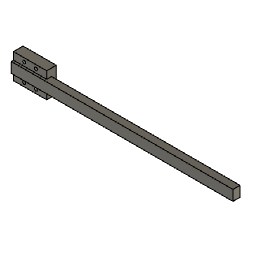
water-suply (Autodesk Fusion 360 archive; units mm, degrees)
design "rail 150mm"
Autodesk Fusion 360 part; units mm, degrees
note: some values were not read from the file. Set by a fixed rule: the direction of a hole.
sketch "스케치1" plane through (0, 0, 0) normal (0, 1, 0) x (1, 0, 0)
  line L0 (0, 0) -> (150, 0) construction
  line L1 (150, 0) -> (150, -17) construction
  line L2 (150, -17) -> (0, -17) construction
  line L3 (0, -17) -> (0, 0) construction
  line L4 (0, -12) -> (150, -12)
  line L5 (150, -12) -> (150, -5)
  line L6 (150, -5) -> (0, -5)
  line L7 (0, -5) -> (0, -12)
  line L8 (35.8106, -17) -> (58.3106, -17)
  line L9 (58.3106, -17) -> (58.3106, 0)
  line L10 (58.3106, 0) -> (35.8106, 0)
  line L11 (35.8106, 0) -> (35.8106, -17)
  line L12 (43.061, -14.5007) -> (51.061, -14.5007) construction
  line L13 (51.061, -14.5007) -> (51.061, -2.5007) construction
  line L14 (51.061, -2.5007) -> (43.061, -2.5007) construction
  line L15 (43.061, -2.5007) -> (43.061, -14.5007) construction
  line L16 (58.3106, -17) -> (35.8106, 0) construction
  line L17 (35.8106, -17) -> (58.3106, 0) construction
  line L18 (47.0606, -8.5) -> (43.061, -2.5007) construction
  line L19 (43.061, -14.5007) -> (47.0606, -8.5) construction
  line L20 (47.0606, -8.5) -> (51.061, -2.5007) construction
  line L21 (51.061, -14.5007) -> (47.0606, -8.5) construction
  point P0 (47.0606, -8.5)
  point P1 (47.0606, -8.5)
  dimension "d1" = 150
  dimension "d2" = 17
  dimension "d3" = 7
  dimension "d4" = 22.5
  dimension "d24" = 8
  dimension "d25" = 12
  constraint horizontal L0
  constraint vertical L1
  constraint horizontal L2
  constraint vertical L3
  constraint coincident L0.start L3.end
  constraint horizontal L4
  constraint vertical L5
  constraint horizontal L6
  constraint vertical L7
  constraint coincident L3 L4.start
  constraint midpoint L3 L7
  constraint horizontal L8
  constraint vertical L9
  constraint horizontal L10
  constraint vertical L11
  constraint coincident L2 L8.start
  constraint collinear L0 L10
  constraint horizontal L12
  constraint vertical L13
  constraint horizontal L14
  constraint vertical L15
  constraint coincident P1 P0
  constraint midpoint L17 P1
  measures "d1" distance of L0.start L0.end
  measures "d2" distance of L0.start L2.end
  measures "d3" distance of L4.start L6.end
  measures "d4" distance of L8.start L8.end
  measures "d24" distance of L12.start L12.end
  measures "d25" distance of L12.start L14.end
extrude "돌출1" add sketch "스케치1" along normal blind 4.8 contours L4 L6 L7 L11 | L4 L6 L9 L11 | L4 L5 L6 L9 makes body 1
copy_body "본체->구성요소1" bodies 1 removing the originals makes body 2 in component "Component'"
extrude "돌출1'" add sketch "스케치1" along normal blind 6.5 from surface at 1.5 separate body contours L4 L6 L9 L11 | L4 L8 L9 L11 | L6 L9 L10 L11 makes body 3 in component "Component"
combine "결합1" operation cut target body 3 tool bodies 2 keep tools in component "Component"
hole "구멍1" at (51.061, 0, 14.5007) at (43.061, 0, 14.5007) at (43.061, 0, 2.5007) at (51.061, 0, 2.5007) direction (0, 1, 0) diameter 2 end through all bodies 3 in component "Component"
component "Component" placed x (1, 0, 0) y (0, 1, 0) z (0, 0, 1) at (-35.8106, 0, 0)
component "Component'" placed x (1, 0, 0) y (0, 1, 0) z (0, 0, 1) at (0, 0, 0)
equation "d21 = -150.00 mm + 22.5 mm"

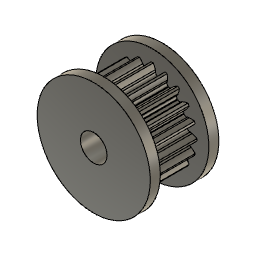
design "gpa20gt2060-a-h4"
description: Spur Gear; Module: 0.611000; Number of Teeth: 20; Pressure Angle: 20.000000; Root Fillet Radius: 0.036000; Clearance: 0.010000; Gear Thickness: 1.030000; Hole Diameter: 0.400000;
Autodesk Fusion 360 part; units mm, degrees
sketch "sketch 251" plane through (0, 0, 0) normal (0, 1, 0) x (1, 0, 0)
  spline S0 degree 3 poles (-6.7198, -0.1571) (-6.4139, -0.333) (-6.1651, -0.4166) (-5.9924, -0.4559) knots 0 0 0 0 1 1 1 1
  spline S1 degree 3 poles (-5.5463, -1.2926) (-5.63, -1.3139) (-5.7122, -1.3421) (-5.84, -1.4181) knots 0 0 0 0 1 1 1 1
  arc A0 (-5.2876, -0.7901) -> (-5.2729, -0.8825) centre (0, 0) ccw
  arc A1 (-5.2876, -0.7901) -> (-5.6742, -0.4846) centre (-5.6436, -0.8433) ccw
  arc A2 (-5.5463, -1.2926) -> (-5.2729, -0.8825) centre (-5.628, -0.942) ccw
  spline S2 degree 3 poles (-6.3424, -2.2259) (-5.9971, -2.2987) (-5.7346, -2.3013) (-5.5582, -2.2853) knots 0 0 0 0 1 1 1 1
  spline S3 degree 3 poles (-5.9924, -0.4559) (-5.8473, -0.4887) (-5.7605, -0.4902) (-5.6742, -0.4846) knots 0 0 0 0 1 1 1 1
  spline S4 degree 3 poles (-5.9924, 0.4559) (-6.1651, 0.4166) (-6.4139, 0.333) (-6.7198, 0.1571) knots 0 0 0 0 1 1 1 1
  arc A3 (-6.7198, 0.1571) -> (-6.7198, -0.1571) centre (0, 0) ccw
  spline S5 degree 3 poles (-5.3441, -4.0769) (-4.9932, -4.0394) (-4.7428, -3.9608) (-4.5799, -3.8911) knots 0 0 0 0 1 1 1 1
  spline S6 degree 3 poles (-3.1534, -5.1159) (-3.0416, -5.0179) (-2.9894, -4.9484) (-2.9432, -4.8754) knots 0 0 0 0 1 1 1 1
  arc A4 (-2.4688, -4.7421) -> (-2.3853, -4.7846) centre (0, 0) ccw
  spline S7 degree 3 poles (-5.5582, -2.2853) (-5.4101, -2.2717) (-5.3271, -2.2463) (-5.2468, -2.2143) knots 0 0 0 0 1 1 1 1
  arc A5 (-3.7273, -4.3057) -> (-3.7471, -3.8133) centre (-3.9994, -4.0701) ccw
  spline S8 degree 3 poles (-2.2853, -5.5582) (-2.3013, -5.7346) (-2.2987, -5.9971) (-2.2259, -6.3424) knots 0 0 0 0 1 1 1 1
  arc A6 (-0.1571, -6.7198) -> (0.1571, -6.7198) centre (0, 0) ccw
  spline S9 degree 3 poles (-3.7273, -4.3057) (-3.7825, -4.3722) (-3.8323, -4.4433) (-3.8911, -4.5799) knots 0 0 0 0 1 1 1 1
  spline S10 degree 3 poles (-0.4559, -5.9924) (-0.4166, -6.1651) (-0.333, -6.4139) (-0.1571, -6.7198) knots 0 0 0 0 1 1 1 1
  spline S11 degree 3 poles (-3.8911, -4.5799) (-3.9608, -4.7428) (-4.0394, -4.9932) (-4.0769, -5.3441) knots 0 0 0 0 1 1 1 1
  spline S12 degree 3 poles (0.1571, -6.7198) (0.333, -6.4139) (0.4166, -6.1651) (0.4559, -5.9924) knots 0 0 0 0 1 1 1 1
  arc A7 (-4.0769, -5.3441) -> (-3.8227, -5.5288) centre (0, 0) ccw
  spline S13 degree 3 poles (-2.2143, -5.2468) (-2.2463, -5.3271) (-2.2717, -5.4101) (-2.2853, -5.5582) knots 0 0 0 0 1 1 1 1
  spline S14 degree 3 poles (1.2926, -5.5463) (1.3139, -5.63) (1.3421, -5.7122) (1.4181, -5.84) knots 0 0 0 0 1 1 1 1
  spline S15 degree 3 poles (0.4559, -5.9924) (0.4887, -5.8473) (0.4902, -5.7605) (0.4846, -5.6742) knots 0 0 0 0 1 1 1 1
  arc A8 (-0.4846, -5.6742) -> (-0.7901, -5.2876) centre (-0.8433, -5.6436) ccw
  spline S16 degree 3 poles (-0.4846, -5.6742) (-0.4902, -5.7605) (-0.4887, -5.8473) (-0.4559, -5.9924) knots 0 0 0 0 1 1 1 1
  arc A9 (-0.8825, -5.2729) -> (-0.7901, -5.2876) centre (0, 0) ccw
  arc A10 (-5.5288, -3.8227) -> (-5.3441, -4.0769) centre (0, 0) ccw
  arc A11 (1.2926, -5.5463) -> (0.8825, -5.2729) centre (0.942, -5.628) ccw
  arc A12 (0.7901, -5.2876) -> (0.8825, -5.2729) centre (0, 0) ccw
  spline S17 degree 3 poles (-5.1159, -3.1534) (-5.2325, -3.2867) (-5.3847, -3.5006) (-5.5288, -3.8227) knots 0 0 0 0 1 1 1 1
  spline S18 degree 3 poles (-5.84, -1.4181) (-5.9921, -1.5089) (-6.2029, -1.6653) (-6.4395, -1.9271) knots 0 0 0 0 1 1 1 1
  arc A13 (-2.4688, -4.7421) -> (-2.9432, -4.8754) centre (-2.635, -5.0614) ccw
  spline S19 degree 3 poles (-3.8227, -5.5288) (-3.5006, -5.3847) (-3.2867, -5.2325) (-3.1534, -5.1159) knots 0 0 0 0 1 1 1 1
  arc A14 (-4.8754, -2.9432) -> (-4.7421, -2.4688) centre (-5.0614, -2.635) ccw
  arc A15 (-2.2259, -6.3424) -> (-1.9271, -6.4395) centre (0, 0) ccw
  spline S20 degree 3 poles (-4.5799, -3.8911) (-4.4433, -3.8323) (-4.3722, -3.7825) (-4.3057, -3.7273) knots 0 0 0 0 1 1 1 1
  arc A16 (-0.8825, -5.2729) -> (-1.2926, -5.5463) centre (-0.942, -5.628) ccw
  spline S21 degree 3 poles (-1.4181, -5.84) (-1.3421, -5.7122) (-1.3139, -5.63) (-1.2926, -5.5463) knots 0 0 0 0 1 1 1 1
  arc A17 (0.7901, -5.2876) -> (0.4846, -5.6742) centre (0.8433, -5.6436) ccw
  spline S22 degree 3 poles (1.4181, -5.84) (1.5089, -5.9921) (1.6653, -6.2029) (1.9271, -6.4395) knots 0 0 0 0 1 1 1 1
  spline S23 degree 3 poles (-4.8754, -2.9432) (-4.9484, -2.9894) (-5.0179, -3.0416) (-5.1159, -3.1534) knots 0 0 0 0 1 1 1 1
  arc A18 (-4.7846, -2.3853) -> (-4.7421, -2.4688) centre (0, 0) ccw
  arc A19 (-3.8133, -3.7471) -> (-4.3057, -3.7273) centre (-4.0701, -3.9994) ccw
  arc A20 (-2.2143, -5.2468) -> (-2.3853, -4.7846) centre (-2.546, -5.1068) ccw
  spline S24 degree 3 poles (-1.9271, -6.4395) (-1.6653, -6.2029) (-1.5089, -5.9921) (-1.4181, -5.84) knots 0 0 0 0 1 1 1 1
  arc A21 (-6.4395, -1.9271) -> (-6.3424, -2.2259) centre (0, 0) ccw
  arc A22 (-4.7846, -2.3853) -> (-5.2468, -2.2143) centre (-5.1068, -2.546) ccw
  arc A23 (-3.8133, -3.7471) -> (-3.7471, -3.8133) centre (0, 0) ccw
  arc A24 (5.3441, -4.0769) -> (5.5288, -3.8227) centre (0, 0) ccw
  arc A25 (2.3853, -4.7846) -> (2.4688, -4.7421) centre (0, 0) ccw
  spline S25 degree 3 poles (4.3057, -3.7273) (4.3722, -3.7825) (4.4433, -3.8323) (4.5799, -3.8911) knots 0 0 0 0 1 1 1 1
  spline S26 degree 3 poles (5.1159, -3.1534) (5.0179, -3.0416) (4.9484, -2.9894) (4.8754, -2.9432) knots 0 0 0 0 1 1 1 1
  arc A26 (1.9271, -6.4395) -> (2.2259, -6.3424) centre (0, 0) ccw
  arc A27 (4.7421, -2.4688) -> (4.8754, -2.9432) centre (5.0614, -2.635) ccw
  arc A28 (5.2468, -2.2143) -> (4.7846, -2.3853) centre (5.1068, -2.546) ccw
  spline S27 degree 3 poles (5.5288, -3.8227) (5.3847, -3.5006) (5.2325, -3.2867) (5.1159, -3.1534) knots 0 0 0 0 1 1 1 1
  arc A29 (2.9432, -4.8754) -> (2.4688, -4.7421) centre (2.635, -5.0614) ccw
  spline S28 degree 3 poles (2.9432, -4.8754) (2.9894, -4.9484) (3.0416, -5.0179) (3.1534, -5.1159) knots 0 0 0 0 1 1 1 1
  arc A30 (3.8227, -5.5288) -> (4.0769, -5.3441) centre (0, 0) ccw
  arc A31 (3.7471, -3.8133) -> (3.8133, -3.7471) centre (0, 0) ccw
  spline S29 degree 3 poles (4.5799, -3.8911) (4.7428, -3.9608) (4.9932, -4.0394) (5.3441, -4.0769) knots 0 0 0 0 1 1 1 1
  arc A32 (4.3057, -3.7273) -> (3.8133, -3.7471) centre (4.0701, -3.9994) ccw
  spline S30 degree 3 poles (3.1534, -5.1159) (3.2867, -5.2325) (3.5006, -5.3847) (3.8227, -5.5288) knots 0 0 0 0 1 1 1 1
  spline S31 degree 3 poles (4.0769, -5.3441) (4.0394, -4.9932) (3.9608, -4.7428) (3.8911, -4.5799) knots 0 0 0 0 1 1 1 1
  arc A33 (4.7421, -2.4688) -> (4.7846, -2.3853) centre (0, 0) ccw
  arc A34 (3.7471, -3.8133) -> (3.7273, -4.3057) centre (3.9994, -4.0701) ccw
  spline S32 degree 3 poles (3.8911, -4.5799) (3.8323, -4.4433) (3.7825, -4.3722) (3.7273, -4.3057) knots 0 0 0 0 1 1 1 1
  spline S33 degree 3 poles (2.2259, -6.3424) (2.2987, -5.9971) (2.3013, -5.7346) (2.2853, -5.5582) knots 0 0 0 0 1 1 1 1
  arc A35 (2.3853, -4.7846) -> (2.2143, -5.2468) centre (2.546, -5.1068) ccw
  spline S34 degree 3 poles (2.2853, -5.5582) (2.2717, -5.4101) (2.2463, -5.3271) (2.2143, -5.2468) knots 0 0 0 0 1 1 1 1
  circle A36 centre (0, 0) radius 2
  spline S35 degree 3 poles (5.2468, -2.2143) (5.3271, -2.2463) (5.4101, -2.2717) (5.5582, -2.2853) knots 0 0 0 0 1 1 1 1
  spline S36 degree 3 poles (-5.84, 1.4181) (-5.7122, 1.3421) (-5.63, 1.3139) (-5.5463, 1.2926) knots 0 0 0 0 1 1 1 1
  arc A37 (-4.7421, 2.4688) -> (-4.8754, 2.9432) centre (-5.0614, 2.635) ccw
  arc A38 (-6.3424, 2.2259) -> (-6.4395, 1.9271) centre (0, 0) ccw
  spline S37 degree 3 poles (-5.5288, 3.8227) (-5.3847, 3.5006) (-5.2325, 3.2867) (-5.1159, 3.1534) knots 0 0 0 0 1 1 1 1
  spline S38 degree 3 poles (-6.4395, 1.9271) (-6.2029, 1.6653) (-5.9921, 1.5089) (-5.84, 1.4181) knots 0 0 0 0 1 1 1 1
  arc A39 (5.2729, -0.8825) -> (5.2876, -0.7901) centre (0, 0) ccw
  arc A40 (5.6742, -0.4846) -> (5.2876, -0.7901) centre (5.6436, -0.8433) ccw
  arc A41 (-5.6742, 0.4846) -> (-5.2876, 0.7901) centre (-5.6436, 0.8433) ccw
  spline S39 degree 3 poles (6.4395, -1.9271) (6.2029, -1.6653) (5.9921, -1.5089) (5.84, -1.4181) knots 0 0 0 0 1 1 1 1
  spline S40 degree 3 poles (5.5582, -2.2853) (5.7346, -2.3013) (5.9971, -2.2987) (6.3424, -2.2259) knots 0 0 0 0 1 1 1 1
  spline S41 degree 3 poles (5.84, -1.4181) (5.7122, -1.3421) (5.63, -1.3139) (5.5463, -1.2926) knots 0 0 0 0 1 1 1 1
  arc A42 (5.2729, -0.8825) -> (5.5463, -1.2926) centre (5.628, -0.942) ccw
  spline S42 degree 3 poles (-5.6742, 0.4846) (-5.7605, 0.4902) (-5.8473, 0.4887) (-5.9924, 0.4559) knots 0 0 0 0 1 1 1 1
  arc A43 (-5.2729, 0.8825) -> (-5.2876, 0.7901) centre (0, 0) ccw
  arc A44 (-5.2729, 0.8825) -> (-5.5463, 1.2926) centre (-5.628, 0.942) ccw
  arc A45 (-4.7421, 2.4688) -> (-4.7846, 2.3853) centre (0, 0) ccw
  arc A46 (6.3424, -2.2259) -> (6.4395, -1.9271) centre (0, 0) ccw
  spline S43 degree 3 poles (-5.5582, 2.2853) (-5.7346, 2.3013) (-5.9971, 2.2987) (-6.3424, 2.2259) knots 0 0 0 0 1 1 1 1
  spline S44 degree 3 poles (-5.2468, 2.2143) (-5.3271, 2.2463) (-5.4101, 2.2717) (-5.5582, 2.2853) knots 0 0 0 0 1 1 1 1
  spline S45 degree 3 poles (-5.1159, 3.1534) (-5.0179, 3.0416) (-4.9484, 2.9894) (-4.8754, 2.9432) knots 0 0 0 0 1 1 1 1
  arc A47 (-5.2468, 2.2143) -> (-4.7846, 2.3853) centre (-5.1068, 2.546) ccw
  arc A48 (3.7273, 4.3057) -> (3.7471, 3.8133) centre (3.9994, 4.0701) ccw
  spline S46 degree 3 poles (5.9924, 0.4559) (5.8473, 0.4887) (5.7605, 0.4902) (5.6742, 0.4846) knots 0 0 0 0 1 1 1 1
  arc A49 (4.7846, 2.3853) -> (4.7421, 2.4688) centre (0, 0) ccw
  spline S47 degree 3 poles (3.1534, 5.1159) (3.0416, 5.0179) (2.9894, 4.9484) (2.9432, 4.8754) knots 0 0 0 0 1 1 1 1
  arc A50 (5.2876, 0.7901) -> (5.6742, 0.4846) centre (5.6436, 0.8433) ccw
  arc A51 (5.5288, 3.8227) -> (5.3441, 4.0769) centre (0, 0) ccw
  spline S48 degree 3 poles (3.8911, 4.5799) (3.9608, 4.7428) (4.0394, 4.9932) (4.0769, 5.3441) knots 0 0 0 0 1 1 1 1
  arc A52 (0.8825, 5.2729) -> (0.7901, 5.2876) centre (0, 0) ccw
  arc A53 (-2.3853, 4.7846) -> (-2.4688, 4.7421) centre (0, 0) ccw
  spline S49 degree 3 poles (-2.2259, 6.3424) (-2.2987, 5.9971) (-2.3013, 5.7346) (-2.2853, 5.5582) knots 0 0 0 0 1 1 1 1
  spline S50 degree 3 poles (-2.9432, 4.8754) (-2.9894, 4.9484) (-3.0416, 5.0179) (-3.1534, 5.1159) knots 0 0 0 0 1 1 1 1
  arc A54 (-2.9432, 4.8754) -> (-2.4688, 4.7421) centre (-2.635, 5.0614) ccw
  arc A55 (5.5463, 1.2926) -> (5.2729, 0.8825) centre (5.628, 0.942) ccw
  spline S51 degree 3 poles (-4.3057, 3.7273) (-4.3722, 3.7825) (-4.4433, 3.8323) (-4.5799, 3.8911) knots 0 0 0 0 1 1 1 1
  arc A56 (-0.7901, 5.2876) -> (-0.4846, 5.6742) centre (-0.8433, 5.6436) ccw
  spline S52 degree 3 poles (-4.0769, 5.3441) (-4.0394, 4.9932) (-3.9608, 4.7428) (-3.8911, 4.5799) knots 0 0 0 0 1 1 1 1
  spline S53 degree 3 poles (1.4181, 5.84) (1.3421, 5.7122) (1.3139, 5.63) (1.2926, 5.5463) knots 0 0 0 0 1 1 1 1
  spline S54 degree 3 poles (5.5463, 1.2926) (5.63, 1.3139) (5.7122, 1.3421) (5.84, 1.4181) knots 0 0 0 0 1 1 1 1
  spline S55 degree 3 poles (5.9924, -0.4559) (6.1651, -0.4166) (6.4139, -0.333) (6.7198, -0.1571) knots 0 0 0 0 1 1 1 1
  arc A57 (4.8754, 2.9432) -> (4.7421, 2.4688) centre (5.0614, 2.635) ccw
  spline S56 degree 3 poles (3.8227, 5.5288) (3.5006, 5.3847) (3.2867, 5.2325) (3.1534, 5.1159) knots 0 0 0 0 1 1 1 1
  spline S57 degree 3 poles (6.7198, 0.1571) (6.4139, 0.333) (6.1651, 0.4166) (5.9924, 0.4559) knots 0 0 0 0 1 1 1 1
  spline S58 degree 3 poles (6.3424, 2.2259) (5.9971, 2.2987) (5.7346, 2.3013) (5.5582, 2.2853) knots 0 0 0 0 1 1 1 1
  arc A58 (2.4688, 4.7421) -> (2.3853, 4.7846) centre (0, 0) ccw
  spline S59 degree 3 poles (4.8754, 2.9432) (4.9484, 2.9894) (5.0179, 3.0416) (5.1159, 3.1534) knots 0 0 0 0 1 1 1 1
  arc A59 (2.4688, 4.7421) -> (2.9432, 4.8754) centre (2.635, 5.0614) ccw
  spline S60 degree 3 poles (2.2143, 5.2468) (2.2463, 5.3271) (2.2717, 5.4101) (2.2853, 5.5582) knots 0 0 0 0 1 1 1 1
  arc A60 (4.0769, 5.3441) -> (3.8227, 5.5288) centre (0, 0) ccw
  spline S61 degree 3 poles (5.3441, 4.0769) (4.9932, 4.0394) (4.7428, 3.9608) (4.5799, 3.8911) knots 0 0 0 0 1 1 1 1
  spline S62 degree 3 poles (0.4846, 5.6742) (0.4902, 5.7605) (0.4887, 5.8473) (0.4559, 5.9924) knots 0 0 0 0 1 1 1 1
  arc A61 (0.4846, 5.6742) -> (0.7901, 5.2876) centre (0.8433, 5.6436) ccw
  arc A62 (3.8133, 3.7471) -> (3.7471, 3.8133) centre (0, 0) ccw
  arc A63 (0.1571, 6.7198) -> (-0.1571, 6.7198) centre (0, 0) ccw
  spline S63 degree 3 poles (2.2853, 5.5582) (2.3013, 5.7346) (2.2987, 5.9971) (2.2259, 6.3424) knots 0 0 0 0 1 1 1 1
  spline S64 degree 3 poles (-1.4181, 5.84) (-1.5089, 5.9921) (-1.6653, 6.2029) (-1.9271, 6.4395) knots 0 0 0 0 1 1 1 1
  spline S65 degree 3 poles (5.84, 1.4181) (5.9921, 1.5089) (6.2029, 1.6653) (6.4395, 1.9271) knots 0 0 0 0 1 1 1 1
  spline S66 degree 3 poles (-1.2926, 5.5463) (-1.3139, 5.63) (-1.3421, 5.7122) (-1.4181, 5.84) knots 0 0 0 0 1 1 1 1
  arc A64 (4.7846, 2.3853) -> (5.2468, 2.2143) centre (5.1068, 2.546) ccw
  spline S67 degree 3 poles (1.9271, 6.4395) (1.6653, 6.2029) (1.5089, 5.9921) (1.4181, 5.84) knots 0 0 0 0 1 1 1 1
  spline S68 degree 3 poles (-0.1571, 6.7198) (-0.333, 6.4139) (-0.4166, 6.1651) (-0.4559, 5.9924) knots 0 0 0 0 1 1 1 1
  arc A65 (0.8825, 5.2729) -> (1.2926, 5.5463) centre (0.942, 5.628) ccw
  arc A66 (-1.9271, 6.4395) -> (-2.2259, 6.3424) centre (0, 0) ccw
  arc A67 (6.7198, -0.1571) -> (6.7198, 0.1571) centre (0, 0) ccw
  arc A68 (3.8133, 3.7471) -> (4.3057, 3.7273) centre (4.0701, 3.9994) ccw
  arc A69 (2.2259, 6.3424) -> (1.9271, 6.4395) centre (0, 0) ccw
  arc A70 (5.2876, 0.7901) -> (5.2729, 0.8825) centre (0, 0) ccw
  arc A71 (6.4395, 1.9271) -> (6.3424, 2.2259) centre (0, 0) ccw
  spline S69 degree 3 poles (0.4559, 5.9924) (0.4166, 6.1651) (0.333, 6.4139) (0.1571, 6.7198) knots 0 0 0 0 1 1 1 1
  spline S70 degree 3 poles (5.1159, 3.1534) (5.2325, 3.2867) (5.3847, 3.5006) (5.5288, 3.8227) knots 0 0 0 0 1 1 1 1
  spline S71 degree 3 poles (5.5582, 2.2853) (5.4101, 2.2717) (5.3271, 2.2463) (5.2468, 2.2143) knots 0 0 0 0 1 1 1 1
  spline S72 degree 3 poles (4.5799, 3.8911) (4.4433, 3.8323) (4.3722, 3.7825) (4.3057, 3.7273) knots 0 0 0 0 1 1 1 1
  arc A72 (-1.2926, 5.5463) -> (-0.8825, 5.2729) centre (-0.942, 5.628) ccw
  arc A73 (-0.7901, 5.2876) -> (-0.8825, 5.2729) centre (0, 0) ccw
  spline S73 degree 3 poles (-0.4559, 5.9924) (-0.4887, 5.8473) (-0.4902, 5.7605) (-0.4846, 5.6742) knots 0 0 0 0 1 1 1 1
  spline S74 degree 3 poles (-2.2853, 5.5582) (-2.2717, 5.4101) (-2.2463, 5.3271) (-2.2143, 5.2468) knots 0 0 0 0 1 1 1 1
  spline S75 degree 3 poles (5.6742, -0.4846) (5.7605, -0.4902) (5.8473, -0.4887) (5.9924, -0.4559) knots 0 0 0 0 1 1 1 1
  spline S76 degree 3 poles (3.7273, 4.3057) (3.7825, 4.3722) (3.8323, 4.4433) (3.8911, 4.5799) knots 0 0 0 0 1 1 1 1
  arc A74 (2.2143, 5.2468) -> (2.3853, 4.7846) centre (2.546, 5.1068) ccw
  arc A75 (-2.3853, 4.7846) -> (-2.2143, 5.2468) centre (-2.546, 5.1068) ccw
  arc A76 (-3.7471, 3.8133) -> (-3.8133, 3.7471) centre (0, 0) ccw
  arc A77 (-3.8227, 5.5288) -> (-4.0769, 5.3441) centre (0, 0) ccw
  spline S77 degree 3 poles (-4.5799, 3.8911) (-4.7428, 3.9608) (-4.9932, 4.0394) (-5.3441, 4.0769) knots 0 0 0 0 1 1 1 1
  spline S78 degree 3 poles (-3.8911, 4.5799) (-3.8323, 4.4433) (-3.7825, 4.3722) (-3.7273, 4.3057) knots 0 0 0 0 1 1 1 1
  spline S79 degree 3 poles (-3.1534, 5.1159) (-3.2867, 5.2325) (-3.5006, 5.3847) (-3.8227, 5.5288) knots 0 0 0 0 1 1 1 1
  arc A78 (-4.3057, 3.7273) -> (-3.8133, 3.7471) centre (-4.0701, 3.9994) ccw
  arc A79 (-3.7471, 3.8133) -> (-3.7273, 4.3057) centre (-3.9994, 4.0701) ccw
  arc A80 (-5.3441, 4.0769) -> (-5.5288, 3.8227) centre (0, 0) ccw
extrude "돌출1" add sketch "sketch 251" along normal blind 10.3 in component "Spur Gear (20 teeth)"
sketch "스케치1" plane through (0, 0, 0) normal (0, 1, 0) x (1, 0, 0) in component "Spur Gear (20 teeth)"
  circle A0 centre (0, 0) radius 6.11 construction
cylinder "원통 기본체1" add diameter 17 height 1.5 placed x (1, 0, 0) y (0, 0, -1) z (0, 1, 0) at (0, 0, 0) in component "Spur Gear (20 teeth)"
cylinder "원통 기본체2" add diameter 17 height -1.5 placed x (1, 0, 0) y (0, 0, -1) z (0, 1, 0) at (0, 10.3, 0) in component "Spur Gear (20 teeth)"
hole "구멍1" at (0, 0, 0) direction (0, 1, 0) diameter 4 end through all in component "Spur Gear (20 teeth)"
component "Spur Gear (20 teeth)" placed x (1, 0, 0) y (0, 1, 0) z (0, 0, 1) at (0, 0, 0)
